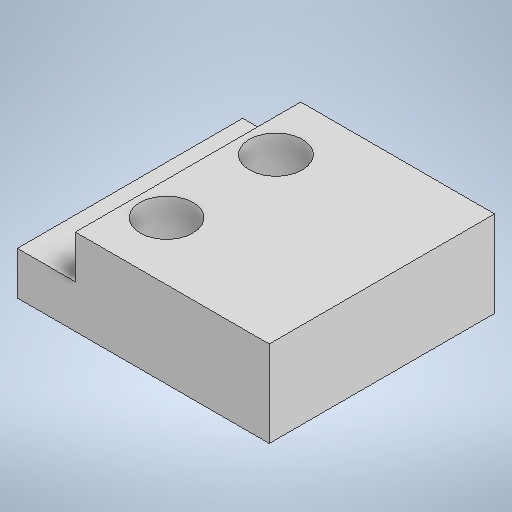
# Autodesk Inventor part: micro usb pin cover
Saved by Autodesk Inventor 2025.1 (Build 291241000, 241)
## iProperties
Created: 2024-09-10
Part Number: micro usb pin cover
Material: Generic
Document SubType Name: Modeling
Designer: clove
Density: 1 g/cm^3
Appearance: Default
Author: clove
Autodesk Inventor part; units mm, degrees
ref_plane "YZ Plane" through (0, 0, 0) normal (1, 0, 0) x (0, 1, 0)
ref_plane "XZ Plane" through (0, 0, 0) normal (0, 1, 0) x (-1, 0, 0)
ref_plane "XY Plane" through (0, 0, 0) normal (0, 0, 1) x (1, 0, 0)
sketch "Sketch1" plane through (0, 0, 0) normal (0, 1, 0) x (-1, 0, 0)
  line L0 (0, 0) -> (15.2, 0)
  line L1 (15.2, 0) -> (15.2, -13.6)
  line L2 (15.2, -13.6) -> (0, -13.6)
  line L3 (0, -13.6) -> (0, 0)
  circle A0 centre (9.7, -3.5) radius 1.6
  circle A1 centre (9.7, -10.1) radius 1.6
  line L4 (9.7, 0) -> (9.7, -13.6) construction
  dimension "d0" = 13.6
  dimension "d1" = 15.2
  dimension "d2" = 3.2
  dimension "d3" = 3.5
  dimension "d4" = 3.5
  dimension "d5" = 5.5
  constraints: 10 end point, 4 point on line, 2 centre point, 2 parallel, 2 perpendicular, 1 equal radius, 1 horizontal
  measures "d0" distance of L2.end L0.start
  measures "d1" distance of L0.start L0.end
  measures "d2" diameter of A0
  measures "d3" distance from line of L2 A1.centre
  measures "d4" distance from line of L0 A0.centre
  measures "d5" distance between parallel lines of L1 L4
extrude "Extrusion1" add sketch "Sketch1" along normal blind 2.6
sketch "Sketch2" plane through (0, 2.6, 0) normal (0, 1, 0) x (1, 0, 0)
  line L0 (0, 0) -> (0, 13.6) projected
  line L1 (0, 13.6) -> (-15.2, 13.6) projected
  line L2 (0, 0) -> (-11.7, 0)
  line L3 (-11.7, 0) -> (-11.7, 13.6)
  line L4 (-11.7, 13.6) -> (0, 13.6)
  line L5 (0, 13.6) -> (0, 0)
  line L6 (-15.2, 13.6) -> (-15.2, 0) projected
  circle A0 centre (-9.7, 10.1) radius 1.6
  circle A1 centre (-9.7, 3.5) radius 1.6
  circle A2 centre (-9.7, 3.5) radius 1.6 projected
  circle A3 centre (-9.7, 10.1) radius 1.6 projected
  point P0 (-15.2, 6.8)
  dimension "d9" = 3.5
  constraints: 8 end point, 4 concentric, 2 centre point, 2 parallel, 1 horizontal, 1 midpoint, 1 perpendicular, 1 point on line
  measures "d9" distance from line of point (-15.2, 6.8) L3
extrude "Extrusion3" add sketch "Sketch2" along normal blind 2.6
body "Solid1"
